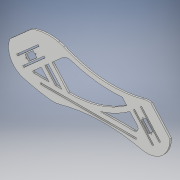
# Autodesk Inventor part: lateral1
Saved by Autodesk Inventor 2019 (Build 230136000, 136)
## iProperties
Created: 2020-02-14
Part Number: lateral1
Material: Genérico
Document SubType Name: Modeling
Designer: Mafer1
Density: 1 g/cm^3
Appearance: Valor por defecto
base_servo: 12.000 mm
altura_servo: 23.000 mm
agujero_servo: 2.000 mm
distancia_agujero_servo: 1.750 mm
soporte: 60.000 mm
largo_base: 200.000 mm
Author: Mafer1
Autodesk Inventor part; units mm, degrees
ref_plane "YZ Plane" through (0, 0, 0) normal (1, 0, 0) x (0, 1, 0)
ref_plane "XZ Plane" through (0, 0, 0) normal (0, 1, 0) x (-1, 0, 0)
ref_plane "XY Plane" through (0, 0, 0) normal (0, 0, 1) x (1, 0, 0)
sketch "Boceto2" plane through (0, 0, 0) normal (0, 0, 1) x (1, 0, 0)
  circle A0 centre (0, 0) radius 42.5
  circle A1 centre (-200, 0) radius 57.5
  circle A2 centre (-250, -5) radius 42.5
  arc A3 (-261.0816, -46.0298) -> (-208.1361, -56.9215) centre (-145.3111, 382.6113) ccw
  arc A4 (-187.598, 56.1466) -> (-283.9285, 20.595) centre (-208.0883, -36.6173) ccw
  arc A5 (-177.0935, 52.7403) -> (-11.2607, 40.9811) centre (-77.5, 282.0461) ccw
  arc A6 (-42.6398, -31) -> (17.7054, 38.6364) centre (-2.2913, -5) ccw
  arc A7 (-13.07, -51.7741) -> (-184.7134, -55.4308) centre (-91.6648, -392.8355) ccw
  dimension "d42" = 85
  dimension "d43" = 200
  dimension "d44" = 115
  dimension "d45" = 85
  dimension "d46" = 50
  dimension "d47" = 5
  dimension "d48" = 444
  dimension "d49" = 95
  dimension "d50" = 250
  dimension "d51" = 350
  dimension "d52" = 5
  dimension "d53" = 48
  dimension "d54" = 31
  constraints: 19 point on circle, 9 tangent, 8 centre point, 1 coincident, 1 horizontal alignment
  measures "d42" diameter of A0
  measures "d43" distance of point (0, 0) A1.centre
  measures "d44" diameter of A1
  measures "d45" diameter of A2
  measures "d46" horizontal distance of A1.centre A2.centre
  measures "d47" vertical distance of A2.centre A1.centre
  measures "d48" radius of A3
  measures "d49" radius of A4
  measures "d50" radius of A5
  measures "d51" radius of A7
  measures "d52" vertical distance of point (0, 0) A6.centre
  measures "d53" radius of A6
  measures "d54" vertical distance of point (0, 0) A6.start
extrude "Extrusión1" add sketch "Boceto2" along normal blind 3.3
sketch "Boceto3" plane through (0, 0, 3.3) normal (0, 0, 1) x (1, 0, 0)
  arc A0 (-177.0935, 52.7403) -> (-11.2607, 40.9811) centre (-77.5, 282.0461) ccw projected
  arc A1 (17.7054, 38.6364) -> (-11.2607, 40.9811) centre (0, 0) ccw projected
  arc A2 (-177.0935, 52.7403) -> (-11.2607, 40.9811) centre (-77.5, 282.0461) ccw projected
  arc A3 (-177.0935, 52.7403) -> (-187.598, 56.1466) centre (-200, 0) ccw projected
  arc A4 (-187.598, 56.1466) -> (-283.9285, 20.595) centre (-208.0883, -36.6173) ccw projected
  arc A5 (-283.9285, 20.595) -> (-261.0816, -46.0298) centre (-250, -5) ccw projected
  arc A6 (-261.0816, -46.0298) -> (-208.1361, -56.9215) centre (-145.3111, 382.6113) ccw projected
  arc A7 (-208.1361, -56.9215) -> (-184.7134, -55.4308) centre (-200, 0) ccw projected
  arc A8 (-13.07, -51.7741) -> (-184.7134, -55.4308) centre (-91.6648, -392.8355) ccw projected
  arc A9 (-13.07, -51.7741) -> (17.7054, 38.6364) centre (-2.2913, -5) ccw projected
  arc A10 (-13.07, -51.7741) -> (17.7054, 38.6364) centre (-2.2913, -5) ccw projected
  arc A11 (17.7054, 38.6364) -> (-11.2607, 40.9811) centre (0, 0) ccw projected
  line L0 (5.6618, 42.1212) -> (45.6618, -2.8788)
  arc A12 (-283.9285, 20.595) -> (-261.0816, -46.0298) centre (-250, -5) ccw projected
  line L1 (-289.2844, 11.2168) -> (-244.2844, 51.2168)
  arc A13 (-187.598, 56.1466) -> (-283.9285, 20.595) centre (-208.0883, -36.6173) ccw projected
  line L2 (-5.3281, 9.3289) -> (9.9523, -7.8615)
  line L3 (9.9523, -7.8615) -> (0.9834, -15.8339)
  line L4 (0.9834, -15.8339) -> (-14.297, 1.3565)
  line L5 (-14.297, 1.3565) -> (-5.3281, 9.3289)
  line L6 (-258.1424, -1.24) -> (-250.17, -10.2089)
  line L7 (-250.17, -10.2089) -> (-232.9796, 5.0714)
  line L8 (-232.9796, 5.0714) -> (-240.9519, 14.0404)
  line L9 (-258.1424, -1.24) -> (-240.9519, 14.0404)
  line L10 (-273.2982, -12.0359) -> (-228.4536, 27.8259)
  line L11 (-230.646, 30.2924) -> (-275.4906, -9.5695)
  line L12 (-262.6683, -23.9945) -> (-217.8238, 15.8674)
  line L13 (-217.8238, 15.8674) -> (-215.6314, 13.4009)
  line L14 (-215.6314, 13.4009) -> (-260.4759, -26.4609)
  line L15 (-260.4759, -26.4609) -> (-262.6683, -23.9945)
  circle A14 centre (-235.6578, 10.7185) radius 1
  circle A15 centre (-255.4641, -6.8871) radius 1
  line L16 (-16.124, 24.4847) -> (23.7378, -20.3599)
  line L17 (23.7378, -20.3599) -> (26.2043, -18.1675)
  line L18 (26.2043, -18.1675) -> (-13.6576, 26.6771)
  line L19 (-13.6576, 26.6771) -> (-16.124, 24.4847)
  line L20 (-28.0826, 13.8548) -> (11.7793, -30.9897)
  line L21 (11.7793, -30.9897) -> (9.3128, -33.1821)
  line L22 (9.3128, -33.1821) -> (-30.549, 11.6624)
  line L23 (-30.549, 11.6624) -> (-28.0826, 13.8548)
  circle A16 centre (-10.9752, 6.6506) radius 1
  circle A17 centre (6.6304, -13.1557) radius 1
  arc A18 (-13.07, -51.7741) -> (-184.7134, -55.4308) centre (-91.6648, -392.8355) ccw projected
  line L24 (-228.4536, 27.8259) -> (-230.646, 30.2924)
  line L25 (-275.4906, -9.5695) -> (-273.2982, -12.0359)
  line L26 (-249.5472, 6.4002) -> (-241.5748, -2.5687) construction
  line L27 (-6.6568, -7.2387) -> (2.3121, 0.7337) construction
  line L28 (-225, -36) -> (-25, -36)
  line L29 (-25, -36) -> (-25, -39.3)
  line L30 (-25, -39.3) -> (-225, -39.3)
  line L31 (-225, -39.3) -> (-225, -36)
  dimension "d59" = 40
  dimension "d60" = 45
  dimension "d61" = 40
  dimension "d62" = 45
  dimension "d65" = 23
  dimension "d66" = 12
  dimension "d68" = 30
  dimension "d69" = 20
  dimension "d70" = 23
  dimension "d71" = 12
  dimension "d73" = 30
  dimension "d74" = 15
  dimension "d75" = 2
  dimension "d76" = 2
  dimension "d77" = 3.3
  dimension "d78" = 3.3
  dimension "d80" = 60
  dimension "d84" = 2
  dimension "d85" = 2
  dimension "d86" = 1.75
  dimension "d87" = 6
  dimension "d88" = 1.75
  dimension "d89" = 6
  dimension "d90" = 2
  dimension "d91" = 2
  dimension "d94" = 3.3
  dimension "d95" = 3.3
  dimension "d96" = 60
  dimension "d97" = 60
  dimension "d98" = 2
  dimension "d99" = 6
  dimension "d100" = 6
  dimension "d101" = 1.75
  dimension "d102" = 1.75
  dimension "d103" = 60
  dimension "d105" = 30
  dimension "d106" = 30
  dimension "d107" = 30
  dimension "d108" = 30
  dimension "d109" = 3.3
  dimension "d110" = 36
  dimension "d111" = 200
  dimension "d112" = 25
  constraints: 64 end point, 19 perpendicular, 4 centre point, 4 midpoint, 4 point on circle, 3 parallel, 1 equal radius, 1 horizontal
  measures "d59" horizontal distance of L0.start L0.end
  measures "d60" vertical distance of L0.start L0.end
  measures "d61" vertical distance of L1.start L1.end
  measures "d62" horizontal distance of L1.start L1.end
  measures "d65" distance of L3.end L4.end
  measures "d66" distance from line of L4 L2.start
  measures "d68" distance between parallel lines of L0 L2
  measures "d69" distance from line of L0.end L3
  measures "d70" distance between parallel lines of L6 L8
  measures "d71" distance between parallel lines of L9 L7
  measures "d73" distance between parallel lines of L9 L1
  measures "d74" distance from line of L6 L1.start
  measures "d75" distance between parallel lines of L9 L10
  measures "d76" distance between parallel lines of L12 L7
  measures "d77" distance between parallel lines of L10 L11
  measures "d78" distance between parallel lines of L12 L14
  measures "d80" distance between parallel lines of L13 L15
  measures "d84" diameter of A14
  measures "d85" diameter of A15
  measures "d86" distance from line of L8 A14.centre
  measures "d87" distance from line of L7 A14.centre
  measures "d88" distance from line of L6 A15.centre
  measures "d89" distance from line of L9 A15.centre
  measures "d90" distance between parallel lines of L2 L16
  measures "d91" distance between parallel lines of L20 L4
  measures "d94" distance between parallel lines of L16 L18
  measures "d95" distance between parallel lines of L22 L20
  measures "d96" distance between parallel lines of L17 L19
  measures "d97" distance between parallel lines of L21 L23
  measures "d98" diameter of A16
  measures "d99" distance from line of L2 A16.centre
  measures "d100" distance from line of A17.centre L2
  measures "d101" distance from line of L5 A16.centre
  measures "d102" distance from line of L3 A17.centre
  measures "d103" distance between parallel lines of L25 L24
  measures "d105" distance between parallel lines of L25 L26
  measures "d106" distance between parallel lines of L27 L17
  measures "d107" distance between parallel lines of L21 L27
  measures "d108" distance between parallel lines of L15 L26
  measures "d109" distance between parallel lines of L30 L28
  measures "d110" distance from line of A1.centre L28
  measures "d111" distance between parallel lines of L29 L31
  measures "d112" horizontal distance of L28.end A1.centre
extrude "Extrusión2" cut sketch "Boceto3" against normal blind 3.3 contours A1 A9 L0 | L1 A5 A4 | L2 L3 L4 L5 | L9 L8 L7 L6 | L25 L11 L24 L10 | L12 L13 L14 L15 | A14 | A15 | L19 L18 L17 L16 | L20 L21 L22 L23 | A16 | A17 | L28 L29 L30 L31
sketch "Sketch4" plane through (0, 0, 3.3) normal (0, 0, 1) x (1, 0, 0)
  arc A0 (-177.0935, 52.7403) -> (-11.2607, 40.9811) centre (-77.5, 282.0461) ccw projected
  line L0 (-225, -36) -> (-25, -36) projected
  arc A1 (-177.0935, 52.7403) -> (-187.598, 56.1466) centre (-200, 0) ccw projected
  arc A2 (-187.598, 56.1466) -> (-244.2844, 51.2168) centre (-208.0883, -36.6173) ccw projected
  line L1 (-207.3674, -26) -> (-239.2844, -26)
  line L2 (45.6618, -2.8788) -> (5.6618, 42.1212) projected
  arc A3 (5.6618, 42.1212) -> (-11.2607, 40.9811) centre (0, 0) ccw projected
  arc A4 (-177.0935, 52.7403) -> (-11.2607, 40.9811) centre (-77.5, 282.0461) ccw projected
  arc A5 (-177.0935, 52.7403) -> (-187.598, 56.1466) centre (-200, 0) ccw projected
  arc A6 (-187.598, 56.1466) -> (-244.2844, 51.2168) centre (-208.0883, -36.6173) ccw projected
  line L3 (-244.2844, 51.2168) -> (-289.2844, 11.2168) projected
  arc A7 (-289.2844, 11.2168) -> (-261.0816, -46.0298) centre (-250, -5) ccw projected
  arc A8 (-261.0816, -46.0298) -> (-208.1361, -56.9215) centre (-145.3111, 382.6113) ccw projected
  arc A9 (-208.1361, -56.9215) -> (-184.7134, -55.4308) centre (-200, 0) ccw projected
  arc A10 (-13.07, -51.7741) -> (-184.7134, -55.4308) centre (-91.6648, -392.8355) ccw projected
  arc A11 (-13.07, -51.7741) -> (45.6618, -2.8788) centre (-2.2913, -5) ccw projected
  line L4 (-232.9796, 5.0714) -> (-250.17, -10.2089) projected
  line L5 (-250.17, -10.2089) -> (-258.1424, -1.24) projected
  line L6 (-258.1424, -1.24) -> (-240.9519, 14.0404) projected
  line L7 (-240.9519, 14.0404) -> (-232.9796, 5.0714) projected
  line L8 (-260.4759, -26.4609) -> (-262.6683, -23.9945) projected
  line L9 (-262.6683, -23.9945) -> (-217.8238, 15.8674) projected
  line L10 (-217.8238, 15.8674) -> (-215.6314, 13.4009) projected
  line L11 (-215.6314, 13.4009) -> (-260.4759, -26.4609) projected
  line L12 (26.2043, -18.1675) -> (23.7378, -20.3599) projected
  line L13 (23.7378, -20.3599) -> (-16.124, 24.4847) projected
  line L14 (-16.124, 24.4847) -> (-13.6576, 26.6771) projected
  line L15 (-13.6576, 26.6771) -> (26.2043, -18.1675) projected
  circle A12 centre (6.6304, -13.1557) radius 1 projected
  circle A13 centre (-255.4641, -6.8871) radius 1 projected
  circle A14 centre (-235.6578, 10.7185) radius 1 projected
  circle A15 centre (-10.9752, 6.6506) radius 1 projected
  line L16 (-30.549, 11.6624) -> (-28.0826, 13.8548) projected
  line L17 (-28.0826, 13.8548) -> (11.7793, -30.9897) projected
  line L18 (11.7793, -30.9897) -> (9.3128, -33.1821) projected
  line L19 (9.3128, -33.1821) -> (-30.549, 11.6624) projected
  line L20 (-230.646, 30.2924) -> (-228.4536, 27.8259) projected
  line L21 (-228.4536, 27.8259) -> (-273.2982, -12.0359) projected
  line L22 (-273.2982, -12.0359) -> (-275.4906, -9.5695) projected
  line L23 (-275.4906, -9.5695) -> (-230.646, 30.2924) projected
  line L24 (-14.297, 1.3565) -> (-5.3281, 9.3289) projected
  line L25 (-5.3281, 9.3289) -> (9.9523, -7.8615) projected
  line L26 (9.9523, -7.8615) -> (0.9834, -15.8339) projected
  line L27 (0.9834, -15.8339) -> (-14.297, 1.3565) projected
  line L28 (-225, -39.3) -> (-225, -36) projected
  line L29 (-225, -36) -> (-25, -36) projected
  line L30 (-25, -36) -> (-25, -39.3) projected
  line L31 (-25, -39.3) -> (-225, -39.3) projected
  line L32 (-215.6314, 13.4009) -> (-260.4759, -26.4609) projected
  arc A16 (-240.7042, -22.2656) -> (-239.2844, -26) centre (-239.2844, -23.8629) ccw
  line L33 (-240.7042, -22.2656) -> (-223.9359, -7.3605)
  line L34 (-223.9359, -7.3605) -> (-207.3674, -26)
  line L35 (-193.9879, -26) -> (-216.4618, -0.7168)
  line L36 (-216.4618, -0.7168) -> (-208.9877, 5.9268)
  line L37 (-208.9877, 5.9268) -> (-180.6083, -26)
  line L38 (-180.6083, -26) -> (-193.9879, -26)
  line L39 (-201.5136, 12.5705) -> (-167.2288, -26)
  line L40 (-201.5136, 12.5705) -> (-180.0872, 31.6162)
  arc A17 (-160.4213, 35.6236) -> (-180.0872, 31.6162) centre (-166.7999, 16.668) ccw
  arc A18 (-160.4213, 35.6236) -> (-54.0967, 23.1015) centre (-77.5, 282.0461) ccw
  line L41 (-54.0967, 23.1015) -> (-44.6998, 12.53)
  arc A19 (-99.3382, -26) -> (-38.0231, 5.0188) centre (-164.0864, 178.0985) ccw
  line L42 (-275.4906, -9.5695) -> (-230.646, 30.2924) projected
  arc A20 (-13.07, -51.7741) -> (45.6618, -2.8788) centre (-2.2913, -5) ccw projected
  line L43 (-99.3382, -26) -> (-29.3382, -26)
  arc A21 (-29.3382, -26) -> (-22.9989, -11.8834) centre (-29.3382, -17.5183) ccw
  line L44 (-38.0231, 5.0188) -> (-22.9989, -11.8834)
  line L45 (9.3128, -33.1821) -> (-30.549, 11.6624) projected
  line L46 (-30.549, 11.6624) -> (-28.0826, 13.8548) projected
  arc A22 (-167.2288, -26) -> (-44.6998, 12.53) centre (-164.0864, 178.0985) ccw
  line L47 (-230.646, 30.2924) -> (-228.4536, 27.8259) projected
  dimension "d113" = 10
  dimension "d114" = 10
  dimension "d115" = 10
  dimension "d117" = 10
  dimension "d119" = 50
  dimension "d121" = 10
  dimension "d126" = 10
  dimension "d129" = 10
  dimension "d130" = 75
  dimension "d131" = 70
  dimension "d132" = 20
  dimension "d136" = 10
  dimension "d139" = 10
  constraints: 24 end point, 12 point on circle, 8 point on line, 6 centre point, 6 tangent, 4 parallel, 2 collinear, 2 concentric, 2 horizontal, 2 perpendicular
  measures "d113" distance between parallel lines of L1 L0
  measures "d114" distance between parallel lines of L35 L34
  measures "d115" distance between parallel lines of L39 L37
  measures "d117" distance between parallel lines of L33 L11
  measures "d119" horizontal distance of A16.centre L3.end
  measures "d121" distance between parallel lines of L37 L35
  measures "d126" radial gap between concentric circles of A18 A0
  measures "d129" distance between parallel lines of L44 L19
  measures "d130" horizontal distance of L2.start A21.centre
  measures "d131" distance of L43.start L43.end
  measures "d132" radius of A17
  measures "d136" radial gap between concentric circles of A22 A19
  measures "d139" distance between parallel lines of L10 L39
extrude "Extrusión5" cut sketch "Sketch4" against normal blind 10 contours L1 A16 L33 L34 | L35 L36 L37 L38 | L40 A17 A18 L41 A22 L39 | A19 L44 A21 L43
equation "\"d45\" = d42"
equation "\"d65\" = altura_servo"
equation "\"d66\" = base_servo"
equation "\"d70\" = d65"
equation "\"d71\" = d66"
equation "\"d78\" = d77"
equation "\"d84\" = agujero_servo"
equation "\"d85\" = d84"
equation "\"d87\" = 0.5 * d71"
equation "\"d88\" = d86"
equation "\"d89\" = 0.5 * d71"
equation "\"d91\" = d90"
equation "\"d95\" = d94"
equation "\"d97\" = d96"
equation "\"d98\" = agujero_servo"
equation "\"d99\" = 0.5 * d66"
equation "\"d100\" = d99"
equation "\"d102\" = d101"
equation "\"soporte\" = 60"
equation "\"largo_base\" = 200"
equation "\"altura_servo\" = 23"
equation "\"base_servo\" = 12"
equation "\"agujero_servo\" = 2"
